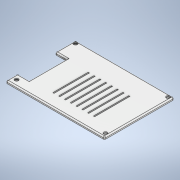
# Autodesk Inventor part: Part3
Saved by Autodesk Inventor 2022 (Build 260153000, 153)
## iProperties
Created: 2023-04-05
Part Number: Part3
Material: ABS Plastic
Document SubType Name: Modeling
Designer: Gibson
Density: 1.06 g/cm^3
Appearance: Smooth - White
Author: Gibson
Autodesk Inventor part; units mm, degrees
ref_plane "YZ Plane" through (0, 0, 0) normal (1, 0, 0) x (0, 1, 0)
ref_plane "XZ Plane" through (0, 0, 0) normal (0, 1, 0) x (-1, 0, 0)
ref_plane "XY Plane" through (0, 0, 0) normal (0, 0, 1) x (1, 0, 0)
sketch "Sketch1" plane through (0, 0, 0) normal (0, 1, 0) x (-1, 0, 0)
  line L0 (22, -33) -> (-148, -33)
  line L1 (22, 2) -> (22, -33)
  line L2 (2, 2) -> (22, 2)
  line L3 (2, 67) -> (2, 2)
  line L4 (22, 67) -> (2, 67)
  line L5 (22, 87) -> (22, 67)
  line L6 (-148, 87) -> (22, 87)
  line L7 (-148, -33) -> (-148, 87)
  circle A0 centre (16.9, -27.9) radius 2.4
  circle A1 centre (13.8, 77) radius 2.4
  arc A2 (-145.3101, 79.6937) -> (-145.3101, 80.5063) centre (-142.9447, 80.1) ccw
  arc A3 (-142.9447, -30.3) -> (-145.3101, -27.4937) centre (-142.9447, -27.9) ccw
  circle A4 centre (-142.9447, -27.9) radius 2.4
  circle A5 centre (-142.9447, 80.1) radius 2.4
  point P0 (0, 0)
  point P1 (22, -33)
  constraints: 16 end point, 6 centre point, 4 point on circle, 1 concentric, 1 point on line
extrude "Extrusion1" add sketch "Sketch1" along normal blind 4
extrude "Extrusion2" add sketch "Sketch1" along normal blind 30 contours A0 | A1 | A5 A2 | A4 A3
fillet "Fillet1" radius 1 4 edges at (-11.4, 30, 77) (-14.5, 30, -27.9) (140.5794, 30, -28.3063) (140.5794, 30, 79.6937)
sketch "Sketch2" plane through (0, 4, 0) normal (0, 1, 0) x (1, 0, 0)
  circle A0 centre (-16.9, 27.9) radius 2.4 projected
  circle A1 centre (142.9447, 27.9) radius 2.4 projected
  circle A2 centre (142.9447, -80.1) radius 2.4 projected
  circle A3 centre (-13.8, -77) radius 2.4 projected
  point P0 (0, 0)
extrude "Extrusion3" cut sketch "Sketch2" along normal through all both and the other way through all
sketch "Sketch3" plane through (0, 0, 0) normal (0, -1, 0) x (1, 0, 0)
  line L0 (37, 65) -> (39, 65)
  line L1 (39, 65) -> (39, 4)
  line L2 (39, 4) -> (37, 4)
  line L3 (37, 4) -> (37, 65)
  point P0 (0, 0)
  constraints: 8 end point, 2 parallel, 1 horizontal, 1 perpendicular
extrude "Extrusion4" cut sketch "Sketch3" against normal through all
pattern_linear "Rectangular Pattern1" count 8 spacing 10 along (1, 0, 0) of "Extrusion4"
sketch "Sketch4" plane through (0, 4, 0) normal (0, 1, 0) x (1, 0, 0)
  circle A0 centre (-16.9, 27.9) radius 2.4 projected
  circle A1 centre (142.9447, 27.9) radius 2.4 projected
  circle A2 centre (142.9447, -80.1) radius 2.4 projected
  circle A3 centre (-13.8, -77) radius 2.4 projected
  circle A4 centre (-16.9, 27.9) radius 3.15
  circle A5 centre (142.9447, 27.9) radius 3.15
  circle A6 centre (142.9447, -80.1) radius 3.15
  circle A7 centre (-13.8, -77) radius 3.15
  point P0 (0, 0)
  dimension "d16" = 0.75
  dimension "d17" = 0.75
  dimension "d18" = 0.75
  dimension "d19" = 0.75
  constraints: 4 centre point
  measures "d16" radial gap between concentric circles of A0 A4
  measures "d17" radial gap between concentric circles of A1 A5
  measures "d18" radial gap between concentric circles of A2 A6
  measures "d19" radial gap between concentric circles of A3 A7
extrude "Extrusion5" cut sketch "Sketch4" against normal blind 1.5 contours A0 | A1 | A2 | A3 | A4 | A5 | A6 | A7
fillet "Fillet2" radius 2 6 edges at (-22, 2, 67) (-22, 2, -33) (-22, 2, 2) (148, 2, -33) (148, 2, 87) (-22, 2, 87)
fillet "Fillet3" radius 2 14 edges at (-2, 4, 34.5) (-21.4142, 4, 1.4142) (-11, 4, 2) (-21.4142, 4, -32.4142) (63, 4, -33) (147.4142, 4, -32.4142) (148, 4, 27) (147.4142, 4, 86.4142) (63, 4, 87) (-21.4142, 4, 86.4142) (-22, 4, 77) (-21.4142, 4, 67.5858) (-11, 4, 67) (-22, 4, -15.5)
body "Solid1"
